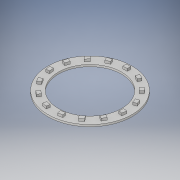
# Autodesk Inventor part: LEDRing
Saved by Autodesk Inventor 2017 (Build 210142000, 142)
## iProperties
Created: 2016-12-05
Part Number: LEDRing
Material: Generic
Document SubType Name: Modeling
Designer: PLTW
Density: 1 g/cm^3
Appearance: Default
Author: PLTW
Autodesk Inventor part; units mm, degrees
ref_plane "YZ Plane" through (0, 0, 0) normal (1, 0, 0) x (0, 1, 0)
ref_plane "XZ Plane" through (0, 0, 0) normal (0, 1, 0) x (-1, 0, 0)
ref_plane "XY Plane" through (0, 0, 0) normal (0, 0, 1) x (1, 0, 0)
sketch "Sketch1" plane through (0, 0, 0) normal (0, 1, 0) x (-1, 0, 0)
  circle A0 centre (0, 0) radius 25.146
  circle A1 centre (0, 0) radius 33.401
  dimension "d0" = 66.802
  dimension "d1" = 50.292
  constraints: 2 centre point, 2 coincident
  measures "d0" diameter of A1
  measures "d1" diameter of A0
extrude "Extrusion1" add sketch "Sketch1" along normal blind 1.524
sketch "Sketch2" plane through (0, 1.524, 0) normal (0, 1, 0) x (1, 0, 0)
  circle A0 centre (0, 0) radius 25.146 projected
  line L0 (-1.75, 27.81) -> (1.75, 27.81)
  line L1 (1.75, 27.81) -> (1.75, 30.61)
  line L2 (1.75, 30.61) -> (-1.75, 30.61)
  line L3 (-1.75, 30.61) -> (-1.75, 27.81)
  line L4 (-1.75, 27.81) -> (1.75, 30.61) construction
  line L5 (1.75, 27.81) -> (-1.75, 30.61) construction
  point P0 (0, 29.21)
  point P1 (0, 29.21)
  dimension "d4" = 3.5
  dimension "d5" = 2.8
  dimension "d6" = 29.21
  constraints: 12 end point, 3 midpoint, 2 parallel, 1 horizontal, 1 perpendicular, 1 vertical alignment
  measures "d4" distance of L1.end L2.end
  measures "d5" distance of L0.end L1.end
  measures "d6" distance of A0.centre point (0, 29.21)
extrude "Extrusion2" add sketch "Sketch2" along normal blind 1.9 contours L3 L2 L1 L0
pattern_circular "Circular Pattern1" count 15 over 360 about axis through (0, 0, 0) along (0, 1, 0) of "Extrusion2"
body "Solid1"
